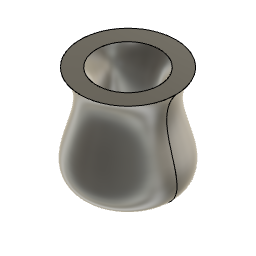
vase (Autodesk Fusion 360 design; units mm, degrees)
Autodesk Fusion 360 part; units mm, degrees
sketch "Sketch1" plane through (0, 0, 0) normal (0, 1, 0) x (1, 0, 0)
  line L0 (0, 0) -> (20, 0)
  spline S0 degree 5 poles (20, 0) (22.1222, -0.4985) (26.1585, -1.5863) (31.5884, -3.4904) (37.5704, -6.5779) (42.9238, -11.3651) (46.1685, -17.0779) (47.4112, -23.6782) (46.9188, -31.0644) (45.1571, -39.0552) (42.6957, -47.4274) (40.1417, -55.9426) (38.0644, -64.3763) (36.9289, -72.5442) (37.011, -80.3345) (38.4413, -87.6918) (40.696, -93.2159) (43.0078, -97.1557) (44.823, -99.6925) (45.799, -100.9385) knots 0 0 0 0 0 0 0.066667 0.133333 0.2 0.266667 0.333333 0.4 0.466667 0.533333 0.6 0.666667 0.733333 0.8 0.866667 0.933333 1 1 1 1 1 1
  line L1 (45.799, -100.9385) -> (30, -100.9385)
  spline S1 degree 5 poles (30, -100.9385) (29.0595, -99.7387) (27.3114, -97.2803) (25.088, -93.4164) (22.9269, -87.9093) (21.5706, -80.4326) (21.5148, -72.3881) (22.6219, -63.8479) (24.6027, -54.9587) (26.9823, -45.9586) (29.1863, -37.1343) (30.6062, -28.7891) (30.673, -21.2059) (28.9244, -14.614) (25.0985, -9.141) (19.0927, -4.8348) (12.5346, -2.3256) (6.643, -0.9625) (2.2859, -0.2827) (0, 0) knots 0 0 0 0 0 0 0.066667 0.133333 0.2 0.266667 0.333333 0.4 0.466667 0.533333 0.6 0.666667 0.733333 0.8 0.866667 0.933333 1 1 1 1 1 1
  point P0 (46.8469, -22.3473)
  point P1 (38.1146, -65.3105)
  point P2 (22.5597, -65.4553)
  point P3 (30, -20)
  constraint coincident L0.start S1.end
  constraint horizontal L0
  constraint horizontal L1
revolve "Revolve1" add sketch "Sketch1" angle 360 about axis through (0, 0, 1.75) along (0, 0, 1)
